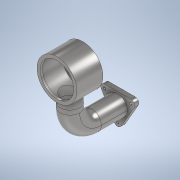
# Autodesk Inventor part: Exhaust_Manifold_2
Saved by Autodesk Inventor 2021 (Build 250183000, 183)
## iProperties
Created: 2021-04-14
Part Number: Exhaust_Manifold_2
Material: Stainless Steel
Document SubType Name: Modeling
Designer: lucia
Density: 8 g/cm^3
Appearance: Semi-Polished
Author: lucia
Autodesk Inventor part; units mm, degrees
ref_plane "YZ Plane" through (0, 0, 0) normal (1, 0, 0) x (0, 1, 0)
ref_plane "XZ Plane" through (0, 0, 0) normal (0, 1, 0) x (-1, 0, 0)
sketch "Sketch1" plane through (0, 0, 0) normal (0, 0, 1) x (1, 0, 0)
  circle A0 centre (0, 0) radius 14.2875
  circle A1 centre (0, 0) radius 17.4625
  circle A2 centre (0, 0) radius 19.05
  circle A3 centre (0, 0) radius 22.8953
  circle A4 centre (0, 0) radius 24.4828
  circle A5 centre (0, 0) radius 27.6578
  circle A6 centre (0, 0) radius 29.2453
  dimension "d0" = 28.575
  dimension "d1" = 34.925
  dimension "d2" = 38.1
  dimension "d207" = 45.7905
  dimension "d208" = 48.9655
  dimension "d209" = 55.3155
  dimension "d210" = 58.4905
  constraints: 7 centre point, 7 coincident
  measures "d0" diameter of A0
  measures "d1" diameter of A1
  measures "d2" diameter of A2
  measures "d207" diameter of A3
  measures "d208" diameter of A4
  measures "d209" diameter of A5
  measures "d210" diameter of A6
extrude "Extrusion1" [suppressed]
sketch "Sketch11" plane through (0, 0, 0) normal (0, 0, 1) x (1, 0, 0)
  circle A0 centre (0, 0) radius 25.908
  circle A1 centre (-38.1, -66.04) radius 12.7
  circle A2 centre (-38.1, -66.04) radius 14.732
  circle A3 centre (-38.1, -66.04) radius 15.748
  line L0 (-38.1, -66.04) -> (-49.1429, -85.181)
  line L1 (-38.1, -66.04) -> (0, 0)
  line L2 (-38.1, -66.04) -> (-49.1551, -46.9061)
  line L3 (-38.1, -66.04) -> (-16.002, -66.0329)
  circle A4 centre (-49.1429, -85.181) radius 1.9844
  circle A5 centre (-49.1551, -46.9061) radius 1.9844
  circle A6 centre (-16.002, -66.0329) radius 1.9844
  circle A7 centre (-16.002, -66.0329) radius 5.5563
  circle A8 centre (-49.1429, -85.181) radius 5.5563
  circle A9 centre (-49.1551, -46.9061) radius 5.5563
  line L4 (-54.6991, -85.1827) -> (-54.7114, -46.9079)
  line L5 (-46.3632, -89.9919) -> (-13.2223, -70.8439)
  line L6 (-13.2254, -61.2202) -> (-46.3785, -42.0934)
  line L7 (0, 0) -> (0, -25.908)
  circle A10 centre (16.002, -66.0329) radius 1.9844
  circle A11 centre (49.1551, -46.9061) radius 1.9844
  circle A12 centre (49.1429, -85.181) radius 1.9844
  line L8 (0, 0) -> (-41.3682, 23.8663)
  line L9 (0, 0) -> (24.0327, 41.6566)
  line L10 (0, 0) -> (61.3648, -35.4028)
  dimension "d137" = 51.816
  dimension "d154" = 0
  dimension "d155" = 360
  dimension "d138" = 38.1
  dimension "d139" = 66.04
  dimension "d140" = 25.4
  dimension "d141" = 29.464
  dimension "d142" = 31.496
  dimension "d143" = 22.098
  dimension "d144" = 120
  dimension "d145" = 120
  dimension "d146" = 22.098
  dimension "d147" = 22.098
  dimension "d148" = 3.9688
  dimension "d149" = 3.9688
  dimension "d150" = 3.9688
  dimension "d151" = 11.1125
  dimension "d152" = 11.1125
  dimension "d153" = 11.1125
  dimension "d159" = 90
  dimension "d160" = 90
  dimension "d161" = 180
  constraints: 22 end point, 12 centre point, 11 coincident, 6 point on circle, 6 tangent, 3 symmetric about line, 1 collinear, 1 vertical, 1 vertical alignment, 8 other
  measures "d138" horizontal distance of point (0, 0) point (-38.1, -66.04)
  measures "d139" vertical distance of point (0, 0) point (-38.1, -66.04)
  measures "d140" diameter of A1
  measures "d141" diameter of A2
  measures "d142" diameter of A3
  measures "d143" distance of L0.start L0.end
  measures "d144" angle of L0 L3
  measures "d145" angle of L0 L2
  measures "d146" distance of L0.start L2.end
  measures "d147" distance of L0.start L3.end
  measures "d148" diameter of A5
  measures "d149" diameter of A6
  measures "d150" diameter of A4
  measures "d151" diameter of A8
  measures "d152" diameter of A7
  measures "d153" diameter of A9
  measures "d159" angle of L8 L1
  measures "d160" angle of L1 L10
  measures "d161" angle of L9 L1
ref_plane "Work Plane8" through (0, 0, 0) normal (0, 0, -1) x (-0.8661856, 0.4997225, 0)
sketch "Sketch12" plane through (0, 0, 0) normal (0, 0, -1) x (-0.8661856, 0.4997225, 0)
  circle A0 centre (0, 0) radius 25.908
  circle A1 centre (-38.1, -66.04) radius 12.7
  circle A2 centre (-38.1, -66.04) radius 14.732
  circle A3 centre (-38.1, -66.04) radius 15.748
  line L0 (-38.1, -66.04) -> (-49.1429, -85.181)
  line L1 (-38.1, -66.04) -> (0, 0)
  line L2 (-38.1, -66.04) -> (-49.1551, -46.9061)
  line L3 (-38.1, -66.04) -> (-16.002, -66.0329)
  circle A4 centre (-49.1429, -85.181) radius 1.9844
  circle A5 centre (-49.1551, -46.9061) radius 1.9844
  circle A6 centre (-16.002, -66.0329) radius 1.9844
  circle A7 centre (-16.002, -66.0329) radius 5.5563
  circle A8 centre (-49.1429, -85.181) radius 5.5563
  circle A9 centre (-49.1551, -46.9061) radius 5.5563
  line L4 (-54.6991, -85.1827) -> (-54.7114, -46.9079)
  line L5 (-46.3632, -89.9919) -> (-13.2223, -70.8439)
  line L6 (-13.2254, -61.2202) -> (-46.3785, -42.0934)
  line L7 (0, 0) -> (0, -25.908)
  circle A10 centre (16.002, -66.0329) radius 1.9844
  circle A11 centre (49.1551, -46.9061) radius 1.9844
  circle A12 centre (49.1429, -85.181) radius 1.9844
  dimension "d162" = 51.816
  dimension "d179" = 0
  dimension "d180" = 360
  dimension "d163" = 38.1
  dimension "d164" = 66.04
  dimension "d165" = 25.4
  dimension "d166" = 29.464
  dimension "d167" = 31.496
  dimension "d168" = 22.098
  dimension "d169" = 120
  dimension "d170" = 120
  dimension "d171" = 22.098
  dimension "d172" = 22.098
  dimension "d173" = 3.9688
  dimension "d174" = 3.9688
  dimension "d175" = 3.9688
  dimension "d176" = 11.1125
  dimension "d177" = 11.1125
  dimension "d178" = 11.1125
  constraints: 16 end point, 12 centre point, 11 coincident, 6 point on circle, 6 tangent, 3 symmetric about line, 1 collinear, 1 vertical, 1 vertical alignment, 8 other
  measures "d163" horizontal distance of point (0, 0) point (-38.1, -66.04)
  measures "d164" vertical distance of point (0, 0) point (-38.1, -66.04)
  measures "d165" diameter of A1
  measures "d166" diameter of A2
  measures "d167" diameter of A3
  measures "d168" distance of L0.start L0.end
  measures "d169" angle of L0 L3
  measures "d170" angle of L0 L2
  measures "d171" distance of L0.start L2.end
  measures "d172" distance of L0.start L3.end
  measures "d173" diameter of A5
  measures "d174" diameter of A6
  measures "d175" diameter of A4
  measures "d176" diameter of A8
  measures "d177" diameter of A7
  measures "d178" diameter of A9
sketch "Sketch13" plane through (0, 0, 0) normal (0, 1, 0) x (-1, 0, 0)
  line L0 (0, 0) -> (0, 19.05)
  circle A0 centre (0, 19.05) radius 14.2875
  circle A1 centre (0, 19.05) radius 12.7
  dimension "d184" = 19.05
  dimension "d185" = 28.575
  dimension "d186" = 25.4
  constraints: 2 centre point, 2 coincident, 2 end point, 1 vertical
  measures "d184" distance of L0.start L0.end
  measures "d185" diameter of A0
  measures "d186" diameter of A1
extrude "Extrusion4" [suppressed]
ref_plane "Work Plane9" through (0, 0, 50.8) normal (0, 0, 1) x (1, 0, 0)
sketch "Sketch16" plane through (0, 0, 50.8) normal (0, 0, 1) x (1, 0, 0)
  circle A0 centre (0, 0) radius 14.2875
  circle A1 centre (0, 0) radius 17.4625
  circle A2 centre (0, 0) radius 19.05
  circle A3 centre (0, 0) radius 22.8953
  circle A4 centre (0, 0) radius 24.4828
  circle A5 centre (0, 0) radius 27.6578
  circle A6 centre (0, 0) radius 29.2453
  dimension "d212" = 28.575
  dimension "d213" = 34.925
  dimension "d214" = 38.1
  dimension "d215" = 45.7905
  dimension "d216" = 48.9655
  dimension "d217" = 55.3155
  dimension "d218" = 58.4905
  constraints: 7 centre point, 7 coincident
  measures "d212" diameter of A0
  measures "d213" diameter of A1
  measures "d214" diameter of A2
  measures "d215" diameter of A3
  measures "d216" diameter of A4
  measures "d217" diameter of A5
  measures "d218" diameter of A6
extrude "Extrusion9" add sketch "Sketch16" along normal blind 38.1 contours A0 | A1 | A2 | A3 | A4 | A5 | A6
sketch "Sketch17" plane through (0, 0, 0) normal (0, 1, 0) x (-1, 0, 0)
  line L0 (0, 0) -> (0, 69.85)
  circle A0 centre (0, 69.85) radius 12.7
  circle A1 centre (0, 69.85) radius 14.2875
  dimension "d221" = 69.85
  dimension "d222" = 25.4
  dimension "d223" = 28.575
  constraints: 2 centre point, 2 coincident, 2 end point, 1 vertical
  measures "d221" distance of L0.start L0.end
  measures "d222" diameter of A0
  measures "d223" diameter of A1
extrude "Extrusion10" add sketch "Sketch17" against normal blind 38.1 contours A0 | A1
shell "Shell2" thickness 1.5875 removed faces 3 at (13.4185, 9.6773, 88.9) at (13.4185, 9.6773, 50.8) at (-4.217, -38.1, 67.6368)
extrude "Extrusion11" add sketch "Sketch16" along normal blind 3.175 contours A5
sketch "Sketch18" plane through (0, 0, 88.9) normal (0, 0, 1) x (1, 0, 0)
  circle A0 centre (0, 0) radius 14.2875
  circle A1 centre (0, 0) radius 17.4625
  circle A2 centre (0, 0) radius 19.05
  circle A3 centre (0, 0) radius 22.8953
  circle A4 centre (0, 0) radius 24.4828
  circle A5 centre (0, 0) radius 27.6578
  circle A6 centre (0, 0) radius 29.2453
  dimension "d229" = 28.575
  dimension "d230" = 34.925
  dimension "d231" = 38.1
  dimension "d232" = 45.7905
  dimension "d233" = 48.9655
  dimension "d234" = 55.3155
  dimension "d235" = 58.4905
  constraints: 7 centre point, 7 coincident
  measures "d229" diameter of A0
  measures "d230" diameter of A1
  measures "d231" diameter of A2
  measures "d232" diameter of A3
  measures "d233" diameter of A4
  measures "d234" diameter of A5
  measures "d235" diameter of A6
extrude "Extrusion12" add sketch "Sketch18" against normal blind 3.175 contours A5
sketch "Sketch19" plane through (0, -38.1, 69.85) normal (0, -1, 0) x (1, 0, 0)
  circle A0 centre (0, 0) radius 12.7
  circle A1 centre (0, 0) radius 14.2875
  point P0 (0, -69.85)
  dimension "d242" = 25.4
  dimension "d243" = 28.575
  constraints: 2 centre point, 1 coincident
  measures "d242" diameter of A0
  measures "d243" diameter of A1
sketch3d "3D Sketch5"
  line L0 (0, -38.1, 69.85) -> (0, -44.4923, 69.85)
  arc A0 (0, -44.4923, 69.85) -> (0, -76.2423, 38.1) centre (0, -44.4923, 38.1) ccw
  line L1 (0, -76.2423, 38.1) -> (0, -76.2423, 0)
  dimension "d239" = 38.1
  dimension "d240" = 31.75
sweep "Sweep3" add profiles "Sketch19" path "3D Sketch5"
extrude "Extrusion13" add sketch "Sketch12" along normal blind 6.35 contours A1 L3 A2 L0 | A1 L1 A2 L3 | L0 A2 L2 A1 | A1 L2 A2 L1 | L3 A3 L0 A2 | A2 L1 A3 L3 | L0 A3 L2 A2 | A2 L2 A3 L1 | L3 A7 L5 A8 L0 A3 | A3 L1 L6 A7 L3 | L0 A8 L4 A9 L2 A3 | A3 L2 A9 L6 L1 | A7 | A8 | A9
extrude "Extrusion14" add sketch "Sketch12" along normal blind 7.366 contours L3 A3 L0 A2 | A2 L1 A3 L3 | L0 A3 L2 A2 | A2 L2 A3 L1
equation "\"d138\" = 9.525 * d156"
equation "\"d139\" = 16.51 * d156"
equation "\"d163\" = 9.525 * d181"
equation "\"d164\" = 16.51 * d181"
equation "\"d3\" = 9.525 * scale"
equation "\"d140\" = 6.35 * d156"
equation "\"d165\" = 6.35 * d181"
equation "\"d36\" = 3.175"
equation "\"d59\" = 3.175"
equation "\"d82\" = 3.175"
equation "\"d104\" = 3.175"
equation "\"d127\" = 3.175"
equation "\"d158\" = 3.175"
equation "\"d183\" = 3.175"
equation "\"scale\" = 4"
equation "\"d156\" = 4"
equation "\"d181\" = 4"
body "Solid1"
